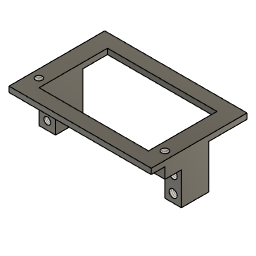
servo_mount v3 (Autodesk Fusion 360 design; units mm, degrees)
Autodesk Fusion 360 part; units mm, degrees
sketch "Sketch1" plane through (0, 0, 0) normal (0, 0, 1) x (1, 0, 0)
  line L0 (26, -17.5) -> (-26, -17.5)
  line L1 (-26, -17.5) -> (-26, 17.5)
  line L2 (-26, 17.5) -> (26, 17.5)
  line L3 (26, 17.5) -> (26, -17.5)
  line L4 (26, -17.5) -> (-26, 17.5) construction
  line L5 (-26, -17.5) -> (26, 17.5) construction
  line L6 (-20, -12.5) -> (20, -12.5)
  line L7 (20, -12.5) -> (20, 12.5)
  line L8 (20, 12.5) -> (-20, 12.5)
  line L9 (-20, 12.5) -> (-20, -12.5)
  line L10 (-20, -12.5) -> (20, 12.5) construction
  line L11 (20, -12.5) -> (-20, 12.5) construction
  dimension "d1" = 52
  dimension "d2" = 35
  dimension "d3" = 40
  dimension "d4" = 25
  constraint horizontal L0
  constraint perpendicular L0 L1
  constraint parallel L0 L2
  constraint parallel L1 L3
  constraint coincident L4 origin
  constraint coincident L5 origin
  constraint horizontal L6
  constraint perpendicular L6 L7
  constraint parallel L6 L8
  constraint parallel L7 L9
  constraint coincident L10 origin
  constraint coincident L11 origin
  measures "d1" distance of L1.end L2.end
  measures "d2" distance of L0.end L1.end
  measures "d3" distance of L7.end L8.end
  measures "d4" distance of L6.end L7.end
extrude "Extrude1" add sketch "Sketch1" along normal blind 2
sketch "Sketch2" plane through (0, 0, 0) normal (0, 0, 1) x (1, 0, 0)
sketch "Sketch3" plane through (0, 0, 0) normal (0, 0, 1) x (1, 0, 0)
  line L0 (-20, -12.5) -> (-26, -12.5)
  line L1 (-26, -12.5) -> (-26, -6.5)
  line L2 (-26, -6.5) -> (-20, -6.5)
  line L3 (-20, -6.5) -> (-20, -12.5)
  dimension "d7" = 6
  constraint horizontal L0
  constraint vertical L1
  constraint horizontal L2
  constraint vertical L3
  measures "d7" distance of L0.start L2.end
extrude "Extrude2" add sketch "Sketch3" against normal blind 4
sketch "Sketch4" plane through (0, 0, 0) normal (0, 0, 1) x (1, 0, 0)
  line L0 (20, -12.5) -> (26, -12.5)
  line L1 (26, -12.5) -> (26, -6.5)
  line L2 (26, -6.5) -> (20, -6.5)
  line L3 (20, -6.5) -> (20, -12.5)
  dimension "d10" = 6
  dimension "d11" = 6
  constraint horizontal L0
  constraint vertical L1
  constraint horizontal L2
  constraint vertical L3
  measures "d10" distance of L0.start L0.end
  measures "d11" distance of L0.start L2.end
extrude "Extrude3" add sketch "Sketch4" against normal blind 4
sketch "Sketch5" plane through (0, 0, 0) normal (0, 0, 1) x (1, 0, 0)
  line L0 (20, -6.5) -> (26, -6.5)
  line L1 (26, -6.5) -> (26, 3.5)
  line L2 (26, 3.5) -> (20, 3.5)
  line L3 (20, 3.5) -> (20, -6.5)
  line L4 (-26, -6.5) -> (-20, -6.5)
  line L5 (-20, -6.5) -> (-20, 3.5)
  line L6 (-20, 3.5) -> (-26, 3.5)
  line L7 (-26, 3.5) -> (-26, -6.5)
  dimension "d14" = 6
  dimension "d15" = 10
  dimension "d16" = 6
  dimension "d17" = 10
  constraint horizontal L0
  constraint vertical L1
  constraint horizontal L2
  constraint vertical L3
  constraint horizontal L4
  constraint vertical L5
  constraint horizontal L6
  constraint vertical L7
  measures "d14" distance of L0.start L0.end
  measures "d15" distance of L0.start L2.end
  measures "d16" distance of L4.start L4.end
  measures "d17" distance of L4.start L6.end
extrude "Extrude4" add sketch "Sketch5" against normal blind 10 contours L0 L1 L2 L3
sketch "Sketch6" plane through (0, 0, 0) normal (0, 0, 1) x (1, 0, 0)
  line L0 (-26, -6.5) -> (-20, -6.5)
  line L1 (-20, -6.5) -> (-20, 3.5)
  line L2 (-20, 3.5) -> (-26, 3.5)
  line L3 (-26, 3.5) -> (-26, -6.5)
  dimension "d20" = 6
  dimension "d21" = 10
  constraint horizontal L0
  constraint vertical L1
  constraint horizontal L2
  constraint vertical L3
  measures "d20" distance of L0.start L0.end
  measures "d21" distance of L0.start L2.end
extrude "Extrude5" add sketch "Sketch6" against normal blind 10
extrude "Extrude6" add 1 faces at (22, 0.1667, -10) along direction (0, 0, -1) blind 6
extrude "Extrude7" add 1 faces at (-24, 0.1667, -10) along direction (0, 0, -1) blind 6
sketch "Sketch7" plane through (0, -6.5, 0) normal (0, -1, 0) x (1, 0, 0)
  line L0 (26, -4) -> (20, -4)
  line L1 (20, -4) -> (20, -16)
  line L2 (20, -16) -> (26, -16)
  line L3 (26, -16) -> (26, -4)
  point P0 (23, -13)
  point P1 (23, -7)
  point P2 (-23, -13)
  point P3 (-23, -7)
hole "Hole1" at (23, -6.5, -13) at (23, -6.5, -7) direction (0, 1, 0) diameter 2.93 depth 10 tip angle 118
thread "Thread1" "ISO Metric profile 3.5 M3.5x0.6 6H"
sketch "Sketch8" plane through (0, -6.5, 0) normal (0, -1, 0) x (1, 0, 0)
  line L0 (-20, -4) -> (-26, -4)
  line L1 (-26, -4) -> (-26, -16)
  line L2 (-26, -16) -> (-20, -16)
  line L3 (-20, -16) -> (-20, -4)
  point P0 (-23, -13)
  point P1 (-23, -7)
hole "Hole2" at (-23, -6.5, -13) at (-23, -6.5, -7) direction (0, 1, 0) diameter 2.529 depth 10 tip angle 118
thread "Thread2" "ISO Metric profile 3.0 M3x0.5 6H"
sketch "Sketch9" plane through (0, 0, -4) normal (0, 0, -1) x (1, 0, 0)
  line L0 (20, 12.5) -> (20, 6.5)
  line L1 (20, 6.5) -> (26, 6.5)
  line L2 (26, 6.5) -> (26, 12.5)
  line L3 (26, 12.5) -> (20, 12.5)
  point P0 (23, 9.5)
  point P1 (-23.051, 9.5)
hole "Hole3" at (-23.051, -9.5, -4) at (23, -9.5, -4) direction (0, 0, 1) diameter 2.529 depth 6 tip angle 118
thread "Thread3" "ISO Metric profile 3.0 M3x0.5 6H"
